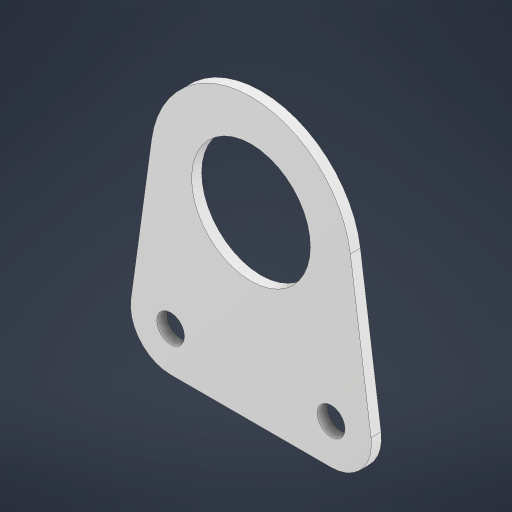
# Autodesk Inventor part: resevoir_mount
Saved by Autodesk Inventor 2024 (Build 280153000, 153)
## iProperties
Created: 2024-01-16
Part Number: resevoir_mount
Material: Acetal Resin, White
Document SubType Name: Modeling
Designer: avere
Density: 1.425 g/cm^3
Appearance: Smooth - White
Author: avere
Autodesk Inventor part; units mm, degrees
ref_plane "YZ Plane" through (0, 0, 0) normal (1, 0, 0) x (0, 1, 0)
ref_plane "XZ Plane" through (0, 0, 0) normal (0, 1, 0) x (-1, 0, 0)
ref_plane "XY Plane" through (0, 0, 0) normal (0, 0, 1) x (1, 0, 0)
sketch "main" plane through (0, 0, 0) normal (0, 0, 1) x (1, 0, 0)
  circle A0 centre (70.448, 399.2567) radius 2.1844
  circle A1 centre (95.848, 399.2567) radius 2.1844
  circle A2 centre (83.148, 421.4817) radius 9.398
  arc A3 (95.848, 392.9067) -> (102.1377, 400.1294) centre (95.848, 399.2567) ccw
  arc A4 (64.1582, 400.1294) -> (70.448, 392.9067) centre (70.448, 399.2567) ccw
  line L0 (95.848, 392.9067) -> (70.448, 392.9067)
  arc A5 (98.8723, 423.6635) -> (67.4236, 423.6635) centre (83.148, 421.4817) ccw
  line L1 (102.1377, 400.1294) -> (98.8723, 423.6635)
  line L2 (67.4236, 423.6635) -> (64.1582, 400.1294)
  point P0 (83.148, 405.9327)
  dimension "d0" = 18.796
  dimension "d1" = 12.7
  dimension "d2" = 12.7
  measures "d0" diameter of A2
  measures "d1" diameter of A3
  measures "d2" diameter of A4
sketch "Sketch1" plane through (0, 0, 0) normal (0, 0, 1) x (1, 0, 0)
  circle A0 centre (0, 0) radius 2.1844
  circle A1 centre (25.4, 0) radius 2.1844
  circle A2 centre (12.7, 22.225) radius 9.398
  arc A3 (25.4, -6.35) -> (31.6897, 0.8727) centre (25.4, 0) ccw
  arc A4 (-6.2897, 0.8727) -> (0, -6.35) centre (0, 0) ccw
  line L0 (25.4, -6.35) -> (0, -6.35)
  arc A5 (28.4244, 24.4068) -> (-3.0244, 24.4068) centre (12.7, 22.225) ccw
  line L1 (31.6897, 0.8727) -> (28.4244, 24.4068)
  line L2 (-3.0244, 24.4068) -> (-6.2897, 0.8727)
  constraints: 1 other
extrude "Extrusion1" add sketch "Sketch1" along normal blind 1.5875
body "Solid1"
